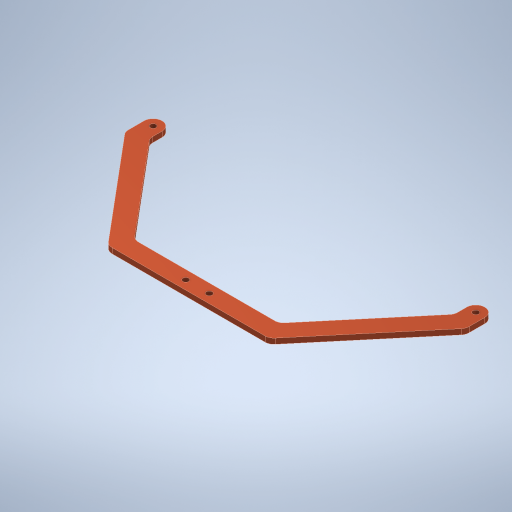
# Autodesk Inventor part: Claw1
Saved by Autodesk Inventor 2023 (Build 270158000, 158)
## iProperties
Created: 2022-11-29
Part Number: Claw1
Material: Copper, Cast
Document SubType Name: Modeling
Designer: kakik
Density: 8.94 g/cm^3
Appearance: Copper - Satin
Author: kakik
Autodesk Inventor part; units mm, degrees
ref_plane "YZ Plane" through (0, 0, 0) normal (1, 0, 0) x (0, 1, 0)
ref_plane "XZ Plane" through (0, 0, 0) normal (0, 1, 0) x (-1, 0, 0)
ref_plane "XY Plane" through (0, 0, 0) normal (0, 0, 1) x (1, 0, 0)
sketch "Sketch1" plane through (0, 0, 0) normal (0, 1, 0) x (-1, 0, 0)
  line L0 (0, 0) -> (0, 10)
  line L1 (0, 10) -> (42.6685, 10)
  line L2 (0, 0) -> (38.0054, 0)
  line L3 (41.8356, -1.7861) -> (83.8302, -51.8333)
  line L4 (85, -55.0472) -> (85, -60.1449)
  line L5 (90, -65.1449) -> (90, -65.1449)
  line L6 (95, -60.1449) -> (95, -51.4075)
  line L7 (93.8302, -48.1936) -> (46.4987, 8.2139)
  arc A0 (45.5995, 9.2856) -> (44.0674, 10) centre (44.0674, 8) ccw
  arc A1 (41.8356, -1.7861) -> (38.0054, 0) centre (38.0054, -5) ccw
  arc A2 (85, -55.0472) -> (83.8302, -51.8333) centre (80, -55.0472) ccw
  arc A3 (95, -51.4075) -> (93.8302, -48.1936) centre (90, -51.4075) ccw
  arc A4 (46.4987, 8.2139) -> (42.6685, 10) centre (42.6685, 5) ccw
  arc A5 (90, -65.1449) -> (95, -60.1449) centre (90, -60.1449) ccw
  arc A6 (85, -60.1449) -> (90, -65.1449) centre (90, -60.1449) ccw
  point P0 (85, -65.1449)
  point P1 (95, -65.1449)
  point P2 (45, 10)
  point P3 (90, -65.1449)
  dimension "d1" = 130
  dimension "d2" = 140
  dimension "d3" = 45
  dimension "d4" = 50
  dimension "d5" = 10
  dimension "d6" = 10
  dimension "d7" = 10
  dimension "d8" = 2
  dimension "d9" = 5
  constraints: 16 end point, 14 point on circle, 14 tangent, 10 point on line, 7 centre point, 5 equal radius, 3 perpendicular, 1 horizontal, 1 parallel, 1 vertical
  measures "d1" angle of L2 L3
  measures "d2" angle of L3 L4
  measures "d3" distance of L0.end point (45, 10)
  measures "d4" horizontal distance of point (45, 10) point (95, -65.145)
  measures "d5" distance of point (85, -65.145) point (95, -65.145)
  measures "d6" distance of L0.start L0.end
  measures "d7" distance between parallel lines of L3 L7
  measures "d8" radius of A0
  measures "d9" radius of A1
extrude "Extrusion1" add sketch "Sketch1" along normal blind 3
sketch "Sketch2" plane through (0, 3, 0) normal (0, 1, 0) x (1, 0, 0)
  line L0 (0, -10) -> (0, 0) projected
  line L1 (0, -5) -> (-25.3234, -5) construction
  arc A0 (-85, 60.1449) -> (-95, 60.1449) centre (-90, 60.1449) ccw projected
  point P0 (-6.55, -5)
  dimension "d19" = 6.55
  constraints: 2 end point, 1 coincident, 1 horizontal, 1 midpoint, 1 point on line
  measures "d19" distance from line of L0 point (-6.55, -5)
hole "Hole1" at (-6.55, 3, 5) at (-90, 3, -60.1449) direction (0, -1, 0) diameter 3.2 end through all clearance for "Countersunk Flat Head Screw DIN EN ISO 2009" size "M3" standard "DIN"
mirror "Mirror1" about plane through (0, 0, 0) normal (1, 0, 0) of "Extrusion1", "Hole1"
body "Solid1"
